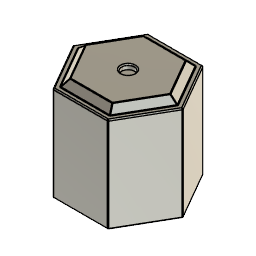
HexQuest Board Piece (Autodesk Fusion 360 design; units mm, degrees)
part number: 2025-09-21-17-01-10-988
part number: 2025-09-25-22-57-21-125
Autodesk Fusion 360 part; units mm, degrees
sketch "Sketch1" plane through (0, 0, 0) normal (0, 0, 1) x (1, 0, 0)
  line L0 (12.7017, -22) -> (25.4034, 0)
  line L1 (25.4034, 0) -> (12.7017, 22)
  line L2 (12.7017, 22) -> (-12.7017, 22)
  line L3 (-12.7017, 22) -> (-25.4034, 0)
  line L4 (-25.4034, 0) -> (-12.7017, -22)
  line L5 (-12.7017, -22) -> (12.7017, -22)
  line L6 (-11.547, -20) -> (11.547, -20)
  line L7 (11.547, -20) -> (23.094, 0)
  line L8 (23.094, 0) -> (11.547, 20)
  line L9 (11.547, 20) -> (-11.547, 20)
  line L10 (-11.547, 20) -> (-23.094, 0)
  line L11 (-23.094, 0) -> (-11.547, -20)
  point P0 (0, 30)
  dimension "d23" = 22
  dimension "d24" = -2
  measures "d23" distance of origin L5
extrude "Extrude1" add sketch "Sketch1" along normal blind 44 contours L0 L1 L2 L3 L4 L5 | L6 L7 L8 L9 L10 L11 makes body 1
extrude "Extrude2" cut sketch "Sketch1" along normal blind 3 contours L6 L7 L8 L9 L10 L11 bodies 1
extrude "Extrude3" add 1 faces at (-3.849, 6.6667, 3) along direction (0, 0, 1) blind 44 on bodies 1 bodies 1
chamfer "Chamfer2" distance 3 angle 45 12 edges at (0, 20, 47) (17.3205, 10, 47) (17.3205, -10, 47) (0, -20, 47) (-17.3205, -10, 47) (-17.3205, 10, 47) (-17.3205, 10, 3) (0, 20, 3) (17.3205, 10, 3) (17.3205, -10, 3) (0, -20, 3) (-17.3205, -10, 3) on bodies 1
move_face "OffsetFaces1" offset -0.1 26 faces at (-3.2718, 5.6669, 3) (-3.2718, 5.6669, 47) (-3.849, 20, 44.0004) (-3.2718, 19.0002, 45.0004) (19.245, 6.6667, 44.0002) (18.0905, 6.6667, 45.0004) (19.245, -6.6667, 44.0004) (14.8188, -12.3335, 45.0004) (-3.849, -20, 44.0002) (-3.2718, -19.0002, 45.0004) (-19.245, -6.6667, 44.0002) (-14.8188, -12.3335, 45.0004) (-15.396, 13.3333, 44.0002) (-18.0905, 6.6667, 45.0004) (14.8188, 12.3335, 1.0004) (19.245, 6.6667, 0.0002) (18.0905, -6.6667, 1.0004) (19.245, -6.6667, 0.0004) (-3.2718, 19.0002, 1.0004) (-3.849, 20, 0.0004) (-14.8188, 12.3335, 1.0004) (-15.396, 13.3333, 0.0002) (-3.2718, -19.0002, 1.0004) (3.849, -20, 0.0004) (-18.0905, -6.6667, 1.0004) (-19.245, -6.6667, 0.0002) on bodies 1
fillet "Fillet6" radius 0.5 54 edges at (10.6282, 18.4086, 45.45) (21.2564, 0, 45.45) (17.198, 9.9293, 44) (14.6866, 8.4793, 46.9) (0, 16.9586, 46.9) (0, 19.8586, 44) (-10.6282, 18.4086, 45.45) (-14.6866, 8.4793, 46.9) (-17.198, 9.9293, 44) (-21.2564, 0, 45.45) (-17.198, -9.9293, 44) (-14.6866, -8.4793, 46.9) (-10.6282, -18.4086, 45.45) (0, -19.8586, 44) (0, -16.9586, 46.9) (10.6282, -18.4086, 45.45) (17.198, -9.9293, 44) (14.6866, -8.4793, 46.9) (-10.7338, -18.5914, 1.55) (-14.7583, -8.5207, 3.1) (-17.443, -10.0707, 0) (-21.4675, 0, 1.55) (-17.443, 10.0707, 0) (-14.7583, 8.5207, 3.1) (-10.7338, 18.5914, 1.55) (0, 20.1414, 0) (0, 17.0414, 3.1) (10.7338, 18.5914, 1.55) (17.443, 10.0707, 0) (14.7583, 8.5207, 3.1) (21.4675, 0, 1.55) (14.7583, -8.5207, 3.1) (17.443, -10.0707, 0) (10.7338, -18.5914, 1.55) (0, -20.1414, 0) (0, -17.0414, 3.1) (19.0526, 11, 44) (19.0526, -11, 44) (25.4034, 0, 22) (19.0526, 11, 0) (19.0526, -11, 0) (0, -22, 0) (12.7017, -22, 22) (-12.7017, -22, 22) (-25.4034, 0, 22) (-19.0526, -11, 0) (-19.0526, 11, 0) (0, 22, 0) (-12.7017, 22, 22) (0, 22, 44) (-19.0526, 11, 44) (0, -22, 44) (-19.0526, -11, 44) (12.7017, 22, 22) on bodies 1
copy_body "Body->Comp1" bodies 1 removing the originals makes body 2 in component "Board Piece"
sketch "Sketch2" plane through (0, 0, 46.9) normal (0, 0, 1) x (-1, 0, 0)
  line L0 (19.3429, 0) -> (9.6715, 16.7515)
  line L1 (9.6715, 16.7515) -> (-9.6715, 16.7515)
  line L2 (-9.6715, 16.7515) -> (-19.3429, 0)
  line L3 (-19.3429, 0) -> (-9.6715, -16.7515)
  line L4 (-9.6715, -16.7515) -> (9.6715, -16.7515)
  line L5 (9.6715, -16.7515) -> (19.3429, 0)
  circle A0 centre (0, 0) radius 2.95
  dimension "d33" = 5.9
  constraint coincident A0.centre origin
  measures "d33" diameter of A0
extrude "Extrude1'" cut sketch "Sketch2" against normal blind 2.2 contours A0 bodies 2 in component "Board Piece"
sketch "Sketch3" plane through (0, 0, 3.1) normal (0, 0, -1) x (1, 0, 0)
  line L0 (9.7193, -16.8343) -> (19.4386, 0)
  line L1 (19.4386, 0) -> (9.7193, 16.8343)
  line L2 (9.7193, 16.8343) -> (-9.7193, 16.8343)
  line L3 (-9.7193, 16.8343) -> (-19.4386, 0)
  line L4 (-19.4386, 0) -> (-9.7193, -16.8343)
  line L5 (-9.7193, -16.8343) -> (9.7193, -16.8343)
  circle A0 centre (0, 0) radius 2.95
  dimension "d38" = 5.9
  constraint coincident A0.centre origin
  measures "d38" diameter of A0
extrude "Extrude2'" cut sketch "Sketch3" against normal blind 2.2 contours A0 bodies 2 in component "Board Piece"
fillet "Fillet2" radius 0.5 2 edges at (-2.7504, -1.0668, 3.1) (2.7504, -1.0668, 46.9) on bodies 2 in component "Board Piece"
component "Board Piece" placed x (1, 0, 0) y (0, 1, 0) z (0, 0, 1) at (0, 0, 0)
